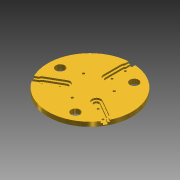
# Autodesk Inventor part: Attachment Point - Female
Saved by Autodesk Inventor 2014 (Build 180170000, 170)
## iProperties
Created: 2014-02-04
Part Number: Attachment Point - Female
Material: Generic
Document SubType Name: Modeling
Designer: Spooner
Density: 1 g/cm^3
Appearance: Gold - Metal
Author: Spooner
Autodesk Inventor part; units mm, degrees
ref_plane "YZ Plane" through (0, 0, 0) normal (1, 0, 0) x (0, 1, 0)
ref_plane "XZ Plane" through (0, 0, 0) normal (0, 1, 0) x (-1, 0, 0)
ref_plane "XY Plane" through (0, 0, 0) normal (0, 0, 1) x (1, 0, 0)
sketch "Sketch1" plane through (0, 0, 0) normal (0, 1, 0) x (-1, 0, 0)
  circle A0 centre (0, 0) radius 60.325
  dimension "d0" = 120.65
  constraints: 1 centre point, 1 coincident
  measures "d0" diameter of A0
extrude "Extrusion1" add sketch "Sketch1" along normal blind 6.35
sketch "Sketch2" plane through (0, 6.35, 0) normal (0, 1, 0) x (1, 0, 0)
  circle A0 centre (0, 0) radius 60.325 projected
  arc A1 (3.81, 50.8) -> (-3.81, 50.8) centre (0, 50.8) ccw
  arc A2 (-3.81, 25.4) -> (3.81, 25.4) centre (0, 25.4) ccw
  line L0 (-3.81, 50.8) -> (-3.81, 25.4)
  line L1 (3.81, 50.8) -> (3.81, 25.4)
  dimension "d3" = 25.4
  dimension "d4" = 7.62
  dimension "d5" = 50.8
  constraints: 4 end point, 4 point on circle, 4 tangent, 2 centre point, 2 vertical alignment, 1 equal radius
  measures "d3" distance of A1.centre A2.centre
  measures "d4" diameter of A2
  measures "d5" distance of A0.centre A1.centre
extrude "Extrusion2" cut sketch "Sketch2" against normal blind 5.08 contours L1 A2 L0 A1
sketch "Sketch3" plane through (0, 6.35, 0) normal (0, 1, 0) x (1, 0, 0)
  line L0 (-3.81, 25.4) -> (-3.81, 50.8) projected
  arc A0 (3.81, 50.8) -> (-3.81, 50.8) centre (0, 50.8) ccw projected
  line L1 (3.81, 50.8) -> (3.81, 25.4) projected
  arc A1 (-3.81, 25.4) -> (3.81, 25.4) centre (0, 25.4) ccw projected
  line L2 (6.35, 25.4) -> (6.35, 50.8)
  arc A2 (6.35, 50.8) -> (-6.35, 50.8) centre (0, 50.8) ccw
  line L3 (-6.35, 50.8) -> (-6.35, 25.4)
  arc A3 (-6.35, 25.4) -> (6.35, 25.4) centre (0, 25.4) ccw
  dimension "d8" = 2.54
  constraints: 4 end point, 4 point on circle, 2 centre point, 3 other
  measures "d8" distance between parallel lines of L2 L1
extrude "Extrusion3" cut sketch "Sketch3" against normal blind 2.54
sketch "Sketch4" plane through (0, 3.81, 0) normal (0, 1, 0) x (1, 0, 0)
  arc A0 (3.81, 50.8) -> (-3.81, 50.8) centre (0, 50.8) ccw projected
  line L0 (-2.54, 67.2746) -> (2.54, 67.2746)
  line L1 (2.54, 67.2746) -> (2.54, 48.8018)
  line L2 (2.54, 48.8018) -> (-2.54, 48.8018)
  line L3 (-2.54, 48.8018) -> (-2.54, 67.2746)
  point P0 (0, 0)
  point P1 (0, 48.8018)
  dimension "d11" = 5.08
  constraints: 8 end point, 2 parallel, 1 horizontal, 1 midpoint, 1 perpendicular, 1 vertical alignment
  measures "d11" distance of L1.end L2.end
extrude "Extrusion4" cut sketch "Sketch4" against normal blind 2.54
sketch "Sketch5" plane through (0, 6.35, 0) normal (0, 1, 0) x (1, 0, 0)
  arc A0 (6.35, 50.8) -> (-6.35, 50.8) centre (0, 50.8) ccw projected
  line L0 (4.7625, 43.4525) -> (-4.7625, 43.4525)
  line L1 (-4.7625, 43.4525) -> (-4.7625, 150.3399)
  line L2 (-4.7625, 150.3399) -> (4.7625, 150.3399)
  line L3 (4.7625, 150.3399) -> (4.7625, 43.4525)
  point P0 (0, 43.4525)
  dimension "d14" = 9.525
  constraints: 8 end point, 2 parallel, 1 horizontal, 1 midpoint, 1 perpendicular, 1 vertical alignment
  measures "d14" distance of L1.end L2.end
extrude "Extrusion5" cut sketch "Sketch5" against normal blind 2.54
sketch "Sketch6" plane through (0, 1.27, 0) normal (0, 1, 0) x (1, 0, 0)
  arc A0 (-2.54, 53.6398) -> (-3.81, 50.8) centre (0, 50.8) ccw projected
  arc A1 (-3.81, 25.4) -> (3.81, 25.4) centre (0, 25.4) ccw projected
  circle A2 centre (0, 50.8) radius 1.524
  circle A3 centre (0, 31.75) radius 1.524
  dimension "d17" = 6.35
  dimension "d18" = 19.05
  dimension "d19" = 3.048
  constraints: 2 centre point, 1 equal radius, 1 vertical alignment
  measures "d17" distance of A1.centre A3.centre
  measures "d18" distance of A2.centre A3.centre
  measures "d19" diameter of A2
extrude "Extrusion6" cut sketch "Sketch6" against normal through all
sketch "Sketch8" plane through (0, 6.35, 0) normal (0, 1, 0) x (1, 0, 0)
  arc A0 (6.35, 50.8) -> (4.7625, 55.0001) centre (0, 50.8) ccw projected
  circle A1 centre (25.4, 38.1) radius 6.35
  dimension "d25" = 12.7
  dimension "d26" = 25.4
  dimension "d27" = 12.7
  constraints: 1 centre point
  measures "d25" diameter of A1
  measures "d26" horizontal distance of A0.centre A1.centre
  measures "d27" vertical distance of A0.centre A1.centre
extrude "Extrusion8" cut sketch "Sketch8" against normal through all
ref_plane "Work Plane1" through (0, 25.4, 25.4) normal (0, 1, 0) x (1, 0, 0)
sketch "Sketch11" plane through (0, 25.4, 25.4) normal (0, 1, 0) x (1, 0, 0)
  circle A0 centre (0, 0) radius 6.35 projected
  circle A1 centre (0, 0) radius 1.7145
  point P0 (0, 25.4)
  dimension "d41" = 3.429
  constraints: 1 centre point, 1 coincident
  measures "d41" diameter of A1
extrude "Extrusion11" cut sketch "Sketch11" against normal through all contours A1
pattern_circular "Circular Pattern2" count 3 over 360 about axis through (0, 0, 0) along (0, 1, 0) of "Extrusion2", "Extrusion3", "Extrusion4", "Extrusion5", "Extrusion6", "Extrusion8", "Extrusion11"
body "Solid1"
